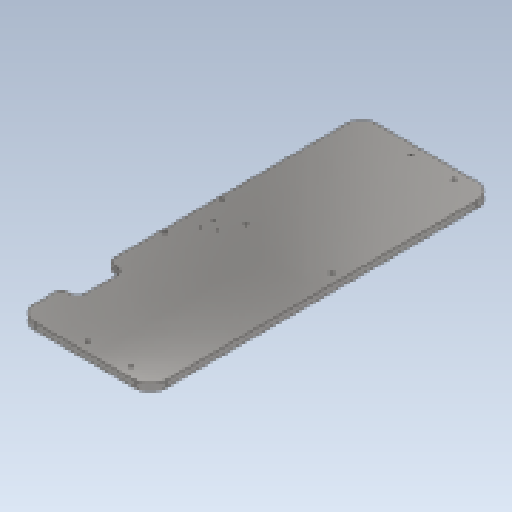
# Autodesk Inventor part: Top_plate
Saved by Autodesk Inventor 2025.2 (Build 292293000, 293)
## iProperties
Created: 2025-02-20
Part Number: Top_plate
Material: Stainless Steel
Document SubType Name: Modeling
Designer: Sergio Quintero
Density: 8 g/cm^3
Appearance: Semi-Polished
Mass: 8245.1 g
Surface Area: 2223.4 cm^2
Volume: 1030.64 cm^3
Author: Sergio Quintero
Autodesk Inventor part; units mm, degrees
ref_plane "YZ Plane" through (0, 0, 0) normal (1, 0, 0) x (0, 1, 0)
ref_plane "XZ Plane" through (0, 0, 0) normal (0, 1, 0) x (-1, 0, 0)
ref_plane "XY Plane" through (0, 0, 0) normal (0, 0, 1) x (1, 0, 0)
sketch "Sketch1" plane through (0, 0, 0) normal (0, 1, 0) x (-1, 0, 0)
  line L0 (-100, -260) -> (100, -260)
  line L1 (100, -260) -> (100, 260)
  line L2 (100, 260) -> (-100, 260)
  line L3 (-100, 260) -> (-100, -260)
  line L4 (-100, -260) -> (100, 260) construction
  line L5 (100, -260) -> (-100, 260) construction
  point P0 (0, 0)
  dimension "d0" = 200
  dimension "d1" = 520
  constraints: 12 end point, 2 midpoint, 2 parallel, 1 horizontal, 1 perpendicular
  measures "d0" distance of L2.end L1.end
  measures "d1" distance of L1.end L0.end
extrude "Extrusion1" add sketch "Sketch1" along normal blind 10
fillet "Fillet1" radius 25 4 edges at (-100, 5, -260) (-100, 5, 260) (100, 5, 260) (100, 5, -260)
sketch "Sketch3" plane through (0, 10, 0) normal (0, 1, 0) x (1, 0, 0)
  line L0 (-75, -260) -> (75, -260) projected
  line L1 (-100, 235) -> (-100, -235) projected
  point P0 (0, 0)
  point P1 (-10, -245)
  point P2 (55, -245)
  dimension "d20" = 15
  dimension "d21" = 90
  dimension "d22" = 65
  dimension "d23" = 15
  measures "d20" distance from line of L0 point (-10, -245)
  measures "d21" distance from line of L1 point (-10, -245)
  measures "d22" distance of point (-10, -245) point (55, -245)
  measures "d23" distance from line of L0 point (55, -245)
hole "Hole2" at (-10, 10, 245) at (55, 10, 245) direction (0, -1, 0) diameter 4.917 end through all thread size "M6x1" class "6H" standard "ISO Metric profile"
mirror "Mirror1" about plane through (0, 0, 0) normal (0, 0, 1) of "Hole2"
sketch "Sketch4" plane through (0, 10, 0) normal (0, 1, 0) x (1, 0, 0)
  line L0 (75, 260) -> (-75, 260) projected
  line L1 (100, -235) -> (100, 235) projected
  point P0 (0, 0)
  point P1 (-45, 30)
  point P2 (85, 30)
  dimension "d31" = 230
  dimension "d32" = 145
  dimension "d33" = 230
  dimension "d34" = 15
  measures "d31" distance from line of L0 point (-45, 30)
  measures "d32" distance from line of L1 point (-45, 30)
  measures "d33" distance from line of L0 point (85, 30)
  measures "d34" distance from line of L1 point (85, 30)
hole "Hole3" at (-45, 10, -30) at (85, 10, -30) direction (0, -1, 0) diameter 4.917 end through all thread size "M6x1" class "6H" standard "ISO Metric profile"
sketch "Sketch12" plane through (0, 0, 0) normal (0, -1, 0) x (1, 0, 0)
  line L0 (0, 0) -> (-38.9736, 0) construction
  line L1 (-100, -235) -> (-100, 235) construction
  point P0 (-74, 10)
  point P1 (-74, -10)
  point P2 (-58, 0)
  dimension "d109" = 10
  dimension "d110" = 26
  dimension "d111" = 16
  constraints: 2 end point, 1 horizontal, 1 point on line, 1 symmetric about line
  measures "d109" distance from line of L0 point (-74, 10)
  measures "d110" distance from line of L1 point (-74, 10)
  measures "d111" horizontal distance of point (-74, 10) point (-58, 0)
hole "Hole8" at (-74, 0, 10) at (-74, 0, -10) at (-58, 0, 0) direction (0, 1, 0) diameter 2.459 end through all thread size "M3x0.5" class "6H" standard "ISO Metric profile"
sketch "Sketch8" plane through (0, 10, 0) normal (0, 1, 0) x (1, 0, 0)
  line L0 (-100, 235) -> (-100, -235) projected
  line L1 (-100, -125) -> (-75, -125)
  line L2 (-75, -125) -> (-75, -195)
  line L3 (-75, -195) -> (-100, -195)
  line L4 (-100, -195) -> (-100, -125)
  line L5 (-75, -260) -> (75, -260) projected
  point P0 (0, 0)
  dimension "d72" = 25
  dimension "d73" = 70
  dimension "d74" = 65
  constraints: 8 end point, 2 parallel, 1 horizontal, 1 perpendicular, 1 point on line
  measures "d72" distance of L2.end L3.end
  measures "d73" distance of L1.end L2.end
  measures "d74" distance between parallel lines of L5 L3
extrude "Extrusion2" cut sketch "Sketch8" against normal blind 10
fillet "Fillet2" radius 10 4 edges at (-100, 5, 125) (-75, 5, 125) (-100, 5, 195) (-75, 5, 195)
sketch "Sketch13" plane through (0, 10, 0) normal (0, 1, 0) x (1, 0, 0)
  line L0 (-100, 235) -> (-100, -115) construction
  line L1 (-100, 0) -> (0, 0) construction
  point P0 (-95, -43)
  point P1 (-95, 43)
  dimension "d119" = 86
  dimension "d120" = 5
  constraints: 2 end point, 1 horizontal, 1 point on line, 1 symmetric about line
  measures "d119" distance of point (-95, 43) point (-95, -43)
  measures "d120" distance from line of L0 point (-95, -43)
hole "Hole9" at (-95, 10, 43) at (-95, 10, -43) direction (0, -1, 0) diameter 4.917 end through all thread size "M6x1" class "6H" standard "ISO Metric profile"
sketch "Sketch9" plane through (0, 10, 0) normal (0, 1, 0) x (1, 0, 0)
  line L0 (-90, 55) -> (-100, 55)
  line L1 (-100, 55) -> (-100, -55)
  line L2 (-100, -55) -> (-90, -55)
  line L3 (-90, -55) -> (-90, 55)
  line L4 (-100, 235) -> (-100, -115) projected
  line L5 (75, 260) -> (-75, 260) projected
  line L6 (0, 0) -> (-100, 0) construction
  dimension "d78" = 10
  dimension "d79" = 110
  dimension "d80" = 0
  constraints: 10 end point, 2 parallel, 2 perpendicular, 1 horizontal, 1 point on line, 1 other
  measures "d78" distance of L2.end L1.end
  measures "d79" distance of L1.end L0.end
  measures "d80" distance between parallel lines of L4 L1
sketch "Sketch10" plane through (0, 10, 0) normal (0, 1, 0) x (1, 0, 0)
  line L0 (-30, 180) -> (-60, 180)
  line L1 (-60, 180) -> (-60, 110)
  line L2 (-60, 110) -> (-30, 110)
  line L3 (-30, 110) -> (-30, 180)
  line L4 (-100, 235) -> (-100, -115) projected
  line L5 (75, 260) -> (-75, 260) projected
  point P0 (0, 0)
  dimension "d85" = 30
  dimension "d86" = 70
  dimension "d87" = 40
  dimension "d88" = 80
  constraints: 8 end point, 2 parallel, 1 horizontal, 1 perpendicular
  measures "d85" distance of L2.end L1.end
  measures "d86" distance of L1.end L0.end
  measures "d87" distance between parallel lines of L4 L1
  measures "d88" distance between parallel lines of L5 L0
sketch "Sketch11" plane through (0, 10, 0) normal (0, 1, 0) x (1, 0, 0)
  line L0 (-100, 235) -> (-100, -115) projected
  line L1 (-100, -205) -> (-100, -235) projected
  line L2 (75, 260) -> (-75, 260) projected
  line L3 (-75, -260) -> (75, -260) projected
  point P0 (0, 0)
  point P1 (-50, 220)
  point P2 (-50, 70)
  point P3 (-50, -80)
  point P4 (-50, -155)
  point P5 (-50, -230)
  dimension "d92" = 50
  dimension "d93" = 50
  dimension "d94" = 50
  dimension "d95" = 50
  dimension "d96" = 50
  dimension "d97" = 40
  dimension "d98" = 190
  dimension "d99" = 180
  dimension "d100" = 105
  dimension "d101" = 30
  measures "d92" distance from line of L0 point (-50, 220)
  measures "d93" distance from line of L0 point (-50, 70)
  measures "d94" distance from line of L0 point (-50, -80)
  measures "d95" distance from line of L0 point (-50, -155)
  measures "d96" distance from line of L1 point (-50, -230)
  measures "d97" distance from line of L2 point (-50, 220)
  measures "d98" distance from line of L2 point (-50, 70)
  measures "d99" distance from line of L3 point (-50, -80)
  measures "d100" distance from line of L3 point (-50, -155)
  measures "d101" distance from line of L3 point (-50, -230)
body "Solid1"
